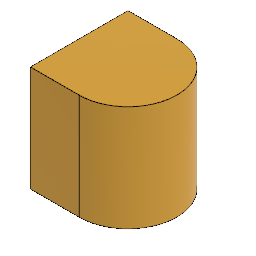
Belt_Tensioner_F01 v1 (Autodesk Fusion 360 design; units mm, degrees)
Autodesk Fusion 360 part; units mm, degrees
sketch "スケッチ1" plane through (0, 0, 0) normal (0, 0, 1) x (1, 0, 0)
  line L0 (0, -3) -> (0, 3)
  line L1 (0, 3) -> (3, 3)
  line L2 (3, 3) -> (3, -3)
  line L3 (3, -3) -> (0, -3)
  arc A0 (3, -3) -> (3, 3) centre (3, 0) ccw
  dimension "d1" = 6
  dimension "d2" = 3
  dimension "d3" = 3
  constraint vertical L0
  constraint perpendicular L0 L1
  constraint perpendicular L1 L2
  constraint perpendicular L2 L3
  constraint midpoint origin L0
  constraint midpoint L2 A0.centre
  measures "d1" distance of L0.start L0.end
  measures "d2" distance of L0.end L1.end
  measures "d3" radius of A0
extrude "押し出し1" add sketch "スケッチ1" along normal blind 6.5
hole "穴1" at (0, 0, 3.25) direction (1, 0, 0) diameter 3.2 depth 2 tip angle 180
